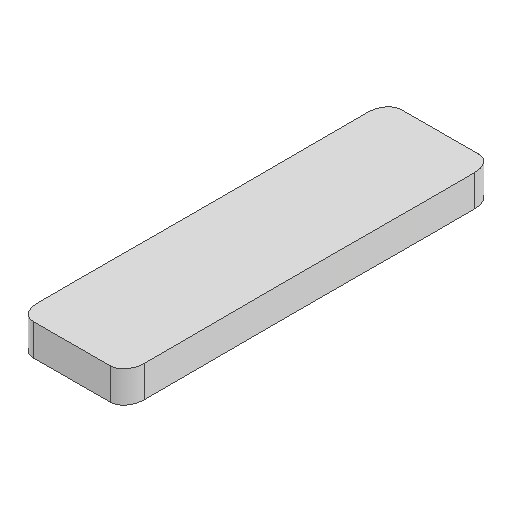
# Autodesk Inventor part: 3DP_PLA_Air_Funnel_Grid
Saved by Autodesk Inventor 2025 (Build 290162010, 162A)
## iProperties
Created: 2024-10-17
Part Number: 3DP_PLA_Air_Funnel_Grid
Material: Generic
Document SubType Name: Modeling
Designer: User
Density: 1 g/cm^3
Appearance: Default
Author: User
Autodesk Inventor part; units mm, degrees
ref_plane "YZ Plane" through (0, 0, 0) normal (1, 0, 0) x (0, 1, 0)
ref_plane "XZ Plane" through (0, 0, 0) normal (0, 1, 0) x (-1, 0, 0)
ref_plane "XY Plane" through (0, 0, 0) normal (0, 0, 1) x (1, 0, 0)
sketch "Sketch1" plane through (0, 0, 0) normal (0, 1, 0) x (-1, 0, 0)
  spline S0 degree 3 poles (-16.4662, -61.0411) (-16.9768, -61.0411) (-17.4763, -60.9416) (-18.4214, -60.5459) (-18.8475, -60.2567) (-19.6563, -59.4765) (-20.0062, -58.969) (-20.4997, -57.9471) (-20.6653, -57.4443) (-20.8869, -56.4029) (-20.9402, -55.861) (-20.9402, -55.3208) knots 0 0 0 0 0.153185 0.153185 0.307403 0.307403 0.489915 0.489915 0.646626 0.646626 0.807788 0.807788 0.807788 0.807788
  line L0 (14.3601, -61.0411) -> (-16.4662, -61.0411)
  spline S1 degree 3 poles (19.0598, -54.8663) (19.0598, -55.9309) (18.8635, -56.9624) (18.1798, -58.6169) (17.7611, -59.261) (16.8631, -60.1665) (16.4105, -60.4909) (15.6597, -60.8212) (15.4064, -60.9035) (14.8872, -61.0136) (14.6244, -61.0411) (14.3601, -61.0411) knots 0 0 0 0 0.319361 0.319361 0.579654 0.579654 0.780076 0.780076 0.876522 0.876522 0.972216 0.972216 0.972216 0.972216
  line L1 (19.0598, 58.2386) -> (19.0598, -54.8663)
  spline S2 degree 3 poles (14.5859, 63.9589) (15.0965, 63.9589) (15.596, 63.8594) (16.541, 63.4638) (16.9672, 63.1745) (17.7759, 62.3943) (18.1258, 61.8869) (18.6193, 60.8649) (18.785, 60.3621) (19.0065, 59.3207) (19.0598, 58.7789) (19.0598, 58.2386) knots 0 0 0 0 0.153185 0.153185 0.307403 0.307403 0.489915 0.489915 0.646626 0.646626 0.807788 0.807788 0.807788 0.807788
  line L2 (-16.2404, 63.9589) -> (14.5859, 63.9589)
  spline S3 degree 3 poles (-20.9402, 57.7841) (-20.9402, 58.8487) (-20.7438, 59.8802) (-20.0601, 61.5347) (-19.6415, 62.1788) (-18.7435, 63.0843) (-18.2909, 63.4088) (-17.5401, 63.739) (-17.2868, 63.8214) (-16.7675, 63.9314) (-16.5048, 63.9589) (-16.2404, 63.9589) knots 0 0 0 0 0.319361 0.319361 0.579654 0.579654 0.780076 0.780076 0.876522 0.876522 0.972216 0.972216 0.972216 0.972216
  line L3 (-20.9402, -55.3208) -> (-20.9402, 57.7841)
  spline S4 degree 3 poles (-17.909, -51.3054) (-18.0017, -34.7045) (-17.8635, -20.3656) (-17.834, 24.2156) (-17.9641, 38.428) (-17.9361, 53.7088) knots 1.062785 1.062785 1.062785 1.062785 6.428499 6.428499 11.956224 11.956224 11.956224 11.956224
  spline S5 degree 3 poles (-13.1357, 60.0284) (-13.638, 60.0242) (-14.1288, 59.921) (-15.0968, 59.519) (-15.5516, 59.2116) (-16.4426, 58.3701) (-16.8406, 57.8065) (-17.4116, 56.6647) (-17.6077, 56.0952) (-17.8699, 54.9224) (-17.935, 54.3146) (-17.9361, 53.7088) knots 0 0 0 0 0.150687 0.150687 0.314293 0.314293 0.517495 0.517495 0.695221 0.695221 0.875662 0.875662 0.875662 0.875662
  spline S6 degree 3 poles (-13.1357, 60.0284) (-9.1116, 60.0623) (-5.089, 60.0828) (3.0852, 60.098) (7.2738, 60.0919) (11.4603, 60.0714) knots 0.852367 0.852367 0.852367 0.852367 2.058296 2.058296 3.311846 3.311846 3.311846 3.311846
  spline S7 degree 3 poles (16.0287, 54.2232) (16.0231, 55.2304) (15.8339, 56.1998) (15.1963, 57.721) (14.8055, 58.3394) (13.9142, 59.2273) (13.4723, 59.5381) (12.7388, 59.8558) (12.4903, 59.9354) (11.9798, 60.0428) (11.7208, 60.0701) (11.4603, 60.0714) knots 0 0 0 0 0.302161 0.302161 0.537205 0.537205 0.71344 0.71344 0.79894 0.79894 0.88426 0.88426 0.88426 0.88426
  spline S8 degree 3 poles (16.0287, 54.2232) (16.1213, 37.6223) (15.9832, 23.2834) (15.9536, -21.2978) (16.0838, -35.5102) (16.0558, -50.791) knots 1.062785 1.062785 1.062785 1.062785 6.428499 6.428499 11.956224 11.956224 11.956224 11.956224
  spline S9 degree 3 poles (11.2554, -57.1106) (11.7576, -57.1063) (12.2484, -57.0032) (13.2164, -56.6011) (13.6712, -56.2938) (14.5622, -55.4523) (14.9602, -54.8887) (15.5312, -53.7469) (15.7273, -53.1774) (15.9896, -52.0046) (16.0547, -51.3968) (16.0558, -50.791) knots 0 0 0 0 0.150687 0.150687 0.314293 0.314293 0.517495 0.517495 0.695221 0.695221 0.875662 0.875662 0.875662 0.875662
  spline S10 degree 3 poles (11.2554, -57.1106) (7.2313, -57.1445) (3.2086, -57.165) (-4.9655, -57.1802) (-9.1542, -57.174) (-13.3406, -57.1536) knots 0.852367 0.852367 0.852367 0.852367 2.058296 2.058296 3.311846 3.311846 3.311846 3.311846
  spline S11 degree 3 poles (-17.909, -51.3054) (-17.9034, -52.3126) (-17.7143, -53.282) (-17.0766, -54.8032) (-16.6858, -55.4216) (-15.7945, -56.3094) (-15.3527, -56.6202) (-14.6192, -56.938) (-14.3706, -57.0176) (-13.8601, -57.1249) (-13.6012, -57.1523) (-13.3406, -57.1536) knots 0 0 0 0 0.302161 0.302161 0.537205 0.537205 0.71344 0.71344 0.79894 0.79894 0.88426 0.88426 0.88426 0.88426
  spline S12 degree 4 poles (15.8558, -50.7906) (15.871, -42.9364) (15.845, -35.0823) (15.7738, -17.2433) (15.7535, 0.5959) (15.7977, 18.9949) (15.869, 37.3938) (15.8769, 45.8081) (15.8287, 54.2221) knots 0 0 0 0 0 0.29917 0.29917 0.679501 0.679501 1 1 1 1 1
  spline S13 degree 5 poles (15.8287, 54.2221) (15.8244, 55.0357) (15.7162, 55.8496) (15.5022, 56.6437) (14.841, 58.1175) (13.6883, 59.2405) (13.0033, 59.664) (12.2284, 59.8677) (11.4593, 59.8714) knots 0 0 0 0 0 0 0.513739 0.513739 0.513739 1 1 1 1 1 1
  spline S14 degree 3 poles (11.4593, 59.8714) (3.2615, 59.9113) (-4.9365, 59.8974) (-13.134, 59.8284) knots 0 0 0 0 1 1 1 1
  spline S15 degree 5 poles (-13.134, 59.8284) (-13.9675, 59.8223) (-14.8062, 59.571) (-15.526, 59.0817) (-16.7178, 57.8452) (-17.4009, 56.2631) (-17.6228, 55.4259) (-17.7348, 54.5665) (-17.7361, 53.7084) knots 0 0 0 0 0 0 0.492985 0.492985 0.492985 1 1 1 1 1 1
  spline S16 degree 4 poles (-17.7361, 53.7084) (-17.7513, 45.8543) (-17.7253, 38.0001) (-17.6542, 20.1611) (-17.6339, 2.322) (-17.6781, -16.0771) (-17.7493, -34.476) (-17.7572, -42.8902) (-17.709, -51.3042) knots 0 0 0 0 0 0.29917 0.29917 0.679501 0.679501 1 1 1 1 1
  spline S17 degree 5 poles (-17.709, -51.3042) (-17.7048, -52.1179) (-17.5966, -52.9318) (-17.3825, -53.7259) (-16.7213, -55.1997) (-15.5686, -56.3226) (-14.8837, -56.7462) (-14.1087, -56.9499) (-13.3396, -56.9536) knots 0 0 0 0 0 0 0.513739 0.513739 0.513739 1 1 1 1 1 1
  spline S18 degree 3 poles (-13.3396, -56.9536) (-5.1419, -56.9935) (3.0561, -56.9795) (11.2537, -56.9106) knots 0 0 0 0 1 1 1 1
  spline S19 degree 5 poles (11.2537, -56.9106) (12.0872, -56.9045) (12.9258, -56.6532) (13.6457, -56.1638) (14.8374, -54.9274) (15.5206, -53.3453) (15.7424, -52.5081) (15.8544, -51.6487) (15.8558, -50.7906) knots 0 0 0 0 0 0 0.492985 0.492985 0.492985 1 1 1 1 1 1
  point P0 (-0.9402, 1.4589)
  dimension "d7" = 0.2
  constraints: 8 end point, 52 other
extrude "Extrusion1" add sketch "Sketch1" along normal blind 10 contours S19 S18 S17 S16 S15 S14 S13 S12
body "Solid1"
